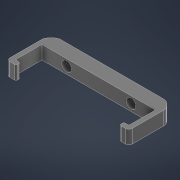
# Autodesk Inventor part: mount_enclosure_coral_dev_board
Saved by Autodesk Inventor 2021 (Build 250183000, 183)
## iProperties
Created: 2021-02-24
Part Number: mount_enclosure_coral_dev_board
Material: ABS Plastic
Document SubType Name: Modeling
Designer: User
Density: 1.06 g/cm^3
Appearance: Smooth - Black
Author: User
Autodesk Inventor part; units mm, degrees
ref_plane "YZ Plane" through (0, 0, 0) normal (1, 0, 0) x (0, 1, 0)
ref_plane "XZ Plane" through (0, 0, 0) normal (0, 1, 0) x (-1, 0, 0)
ref_plane "Work Plane1" through (0, 0, 0) normal (0, 0, 1) x (1, 0, 0)
sketch "base_sketch" plane through (0, 0, 0) normal (0, 0, 1) x (1, 0, 0)
  circle A0 centre (0, -125.6462) radius 1.5 projected
  circle A1 centre (-38, -125.6462) radius 1.5 projected
  line L0 (14.5, -121.6462) -> (-52.5, -121.6462)
  line L1 (-52.5, -121.6462) -> (-52.5, -129.6462)
  line L2 (-52.5, -129.6462) -> (14.5, -129.6462)
  line L3 (14.5, -129.6462) -> (14.5, -121.6462)
  line L4 (-19, -121.6462) -> (-19, -129.6462) construction
  point P0 (0, 0)
  dimension "d1" = 67
  dimension "d4" = 38
  dimension "d5" = 19
  dimension "d6" = 4
  dimension "d7" = 4
  constraints: 10 end point, 2 midpoint, 2 parallel, 1 horizontal, 1 perpendicular
  measures "d1" distance between parallel lines of L1 L3
  measures "d4" distance of A1.centre A0.centre
  measures "d5" distance from line of L4 A0.centre
  measures "d6" distance from line of L0 A0.centre
  measures "d7" distance from line of A0.centre L2
extrude "base" add sketch "base_sketch" along normal blind 8
sketch "holes_bolt_head_sketch" plane through (0, 0, 8) normal (0, 0, 1) x (1, 0, 0)
  circle A0 centre (0, -125.6462) radius 1.5 construction
  circle A1 centre (0, -125.6462) radius 2.9
  circle A2 centre (-38, -125.6462) radius 1.5 construction
  circle A3 centre (-38, -125.6462) radius 2.9
  point P0 (0, 0)
  dimension "d10" = 5.8
  dimension "d11" = 5.8
  constraints: 2 centre point, 2 coincident
  measures "d10" diameter of A3
  measures "d11" diameter of A1
extrude "holes_bolt_head" cut sketch "holes_bolt_head_sketch" against normal blind 3.2
fillet "bolt_head_fillet" radius 0.5 2 edges at (-40.9, -125.6462, 4.8) (-2.9, -125.6462, 4.8)
sketch "walls_sketch" plane through (-52.5, -129.6462, 0) normal (0, -1, 0) x (1, 0, 0)
  line L0 (0, 0) -> (67, 0) projected
  line L1 (67, 0) -> (67, 8) projected
  line L2 (0, 8) -> (67, 8) projected
  line L3 (0, 0) -> (0, 8) projected
  line L4 (67, 8) -> (0, 8) projected
  line L5 (0, 8) -> (0, 23.7)
  line L6 (0, 23.7) -> (3, 23.7)
  line L7 (0, 23.7) -> (3, 23.7) construction
  line L8 (3, 23.7) -> (3, 26.3)
  line L9 (3, 26.3) -> (-2.6, 26.3)
  line L10 (-2.6, 26.3) -> (-2.6, 0)
  line L11 (0, 0) -> (67, 0) projected
  line L12 (-2.6, 0) -> (0, 0)
  line L13 (0, 0) -> (0, 8) projected
  line L14 (33.5, 8) -> (33.5, 0) construction
  line L15 (67, 8) -> (67, 23.7)
  line L16 (67, 23.7) -> (64, 23.7)
  line L17 (64, 23.7) -> (64, 26.3)
  line L18 (64, 26.3) -> (69.6, 26.3)
  line L19 (69.6, 26.3) -> (69.6, 0)
  line L20 (69.6, 0) -> (67, 0)
  point P0 (52.5, 0)
  dimension "d15" = 15.7
  dimension "d16" = 3
  dimension "d17" = 0
  dimension "d18" = 2.6
  dimension "d19" = 2.6
  constraints: 28 end point, 5 perpendicular, 5 symmetric about line, 2 horizontal, 2 midpoint, 1 collinear, 1 vertical
  measures "d15" distance of L2.start L5.end
  measures "d16" distance of L5.end L6.end
  measures "d17" distance between parallel lines of L6 L7
  measures "d18" distance between parallel lines of L3 L10
  measures "d19" distance between parallel lines of L9 L6
extrude "walls" add sketch "walls_sketch" against normal up to surface (8 mm away) contours L12 L10 L9 L8 L6 L5 L3 | L1 L15 L16 L17 L18 L19 L20
fillet "wall_top" radius 2 2 edges at (-55.1, -125.6462, 26.3) (17.1, -125.6462, 26.3)
fillet "wall_tooth" radius 1 4 edges at (-49.5, -125.6462, 26.3) (-49.5, -125.6462, 23.7) (11.5, -125.6462, 23.7) (11.5, -125.6462, 26.3)
chamfer "wall_bottom" distance 4 angle 45 2 edges at (17.1, -125.6462, 0) (-55.1, -125.6462, 0)
fillet "wall_bottom_fillet" radius 4 4 edges at (-55.1, -125.6462, 4) (17.1, -125.6462, 4) (13.1, -125.6462, 0) (-51.1, -125.6462, 0)
fillet "inside" radius 0.5 4 edges at (14.5, -125.6462, 8) (-52.5, -125.6462, 8) (-52.5, -125.6462, 23.7) (14.5, -125.6462, 23.7)
equation "\"d5\" = 0.5 * d4"
equation "\"d7\" = d6"
equation "\"d10\" = d11"
body "Solid1"
